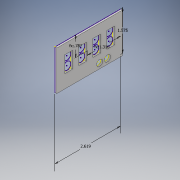
# Autodesk Inventor part: temp_sensor_front_plate
Saved by Autodesk Inventor 2018 (Build 220112000, 112)
## iProperties
Created: 2018-03-26
Part Number: temp_sensor_front_plate
Material: Generic
Document SubType Name: Modeling
Designer: Thomas
Density: 1 g/cm^3
Appearance: Default
Author: Thomas
Autodesk Inventor part; units mm, degrees
ref_plane "YZ Plane" through (0, 0, 0) normal (1, 0, 0) x (0, 1, 0)
ref_plane "XZ Plane" through (0, 0, 0) normal (0, 1, 0) x (-1, 0, 0)
ref_plane "XY Plane" through (0, 0, 0) normal (0, 0, 1) x (1, 0, 0)
sketch "Sketch1" plane through (0, 0, 0) normal (1, 0, 0) x (0, 1, 0)
  line L0 (0, 0) -> (-40, 0)
  line L1 (-40, 0) -> (-40, -66.53)
  line L2 (-40, -66.53) -> (0, -66.53)
  line L3 (0, -66.53) -> (0, 0)
  point P0 (-20, -33.265)
  dimension "d0" = 40
  dimension "d1" = 66.53
  dimension "d13" = 33.265
  dimension "d14" = 20
  constraints: 8 end point, 2 parallel, 1 horizontal, 1 perpendicular
  measures "d0" distance of L2.end L1.end
  measures "d1" distance between parallel lines of L2 L0
  measures "d13" distance from line of point (-20, -33.265) L2
  measures "d14" distance from line of L3 point (-20, -33.265)
extrude "Extrusion1" add sketch "Sketch1" along normal blind 2.04
sketch "Sketch2" plane through (0, 0, 0) normal (1, 0, 0) x (0, 1, 0)
  line L0 (-26.55, -58.615) -> (-9.95, -58.615)
  line L1 (-9.95, -58.615) -> (-9.95, -50.815)
  line L2 (-9.95, -50.815) -> (-26.55, -50.815)
  line L3 (-26.55, -50.815) -> (-26.55, -58.615)
  line L4 (0, -66.53) -> (0, 0) projected
  line L5 (-40, -66.53) -> (0, -66.53) projected
  dimension "d4" = 16.6
  dimension "d5" = 7.8
  dimension "d11" = 9.95
  dimension "d12" = 7.915
  constraints: 8 end point, 2 parallel, 1 horizontal, 1 perpendicular
  measures "d4" distance of L2.end L1.end
  measures "d5" distance between parallel lines of L2 L0
  measures "d11" distance between parallel lines of L1 L4
  measures "d12" distance between parallel lines of L5 L0
extrude "Extrusion2" cut sketch "Sketch2" along normal mid plane 254
pattern_linear "Rectangular Pattern1" count 4 spacing 14.2 along (0, 0, 1) of "Extrusion2"
sketch "Sketch3" plane through (0, 0, 0) normal (1, 0, 0) x (0, 1, 0)
  circle A0 centre (-34.765, -51.34) radius 3.075
  line L0 (-40, -66.53) -> (0, -66.53) projected
  line L1 (-40, 0) -> (-40, -66.53) projected
  point P0 (0, 0)
  dimension "d15" = 6.15
  dimension "d16" = 15.19
  dimension "d17" = 5.235
  constraints: 1 centre point
  measures "d15" diameter of A0
  measures "d16" distance from line of L0 A0.centre
  measures "d17" distance from line of L1 A0.centre
extrude "Extrusion3" cut sketch "Sketch3" along normal up to next
pattern_linear "Rectangular Pattern2" count 2 spacing 8 along (0, 0, 1) of "Extrusion3"
sketch "Sketch4" plane through (0, 0, 0) normal (-1, 0, 0) x (0, 0, 1)
  circle A0 centre (-43.34, -34.765) radius 3.075 projected
  circle A1 centre (-51.34, -34.765) radius 3.075 projected
  line L0 (-8.215, -26.55) -> (-16.015, -26.55) projected
  line L1 (-16.015, -26.55) -> (-16.015, -9.95) projected
  line L2 (-16.015, -9.95) -> (-8.215, -9.95) projected
  line L3 (-8.215, -9.95) -> (-8.215, -26.55) projected
  line L4 (-22.415, -26.55) -> (-30.215, -26.55) projected
  line L5 (-30.215, -26.55) -> (-30.215, -9.95) projected
  line L6 (-30.215, -9.95) -> (-22.415, -9.95) projected
  line L7 (-22.415, -9.95) -> (-22.415, -26.55) projected
  line L8 (-36.615, -26.55) -> (-44.415, -26.55) projected
  line L9 (-44.415, -26.55) -> (-44.415, -9.95) projected
  line L10 (-44.415, -9.95) -> (-36.615, -9.95) projected
  line L11 (-36.615, -9.95) -> (-36.615, -26.55) projected
  line L12 (-50.815, -26.55) -> (-58.615, -26.55) projected
  line L13 (-58.615, -26.55) -> (-58.615, -9.95) projected
  line L14 (-58.615, -9.95) -> (-50.815, -9.95) projected
  line L15 (-50.815, -9.95) -> (-50.815, -26.55) projected
  line L16 (0, 0) -> (0, -40) projected
  line L17 (-66.53, 0) -> (0, 0) projected
  line L18 (-66.53, -40) -> (-66.53, 0) projected
  line L19 (0, -40) -> (-66.53, -40) projected
  circle A2 centre (-54.715, -13.85) radius 3.9
  circle A3 centre (-54.715, -22.65) radius 3.9
  circle A4 centre (-40.515, -13.85) radius 3.9
  circle A5 centre (-40.515, -22.65) radius 3.9
  circle A6 centre (-26.315, -13.85) radius 3.9
  circle A7 centre (-26.315, -22.65) radius 3.9
  circle A8 centre (-12.115, -13.85) radius 3.9
  circle A9 centre (-12.115, -22.65) radius 3.9
  constraints: 24 tangent, 8 centre point
equation "\"d13\" = 0.5 * d1"
equation "\"d14\" = 0.5 * d0"
body "Solid1"
